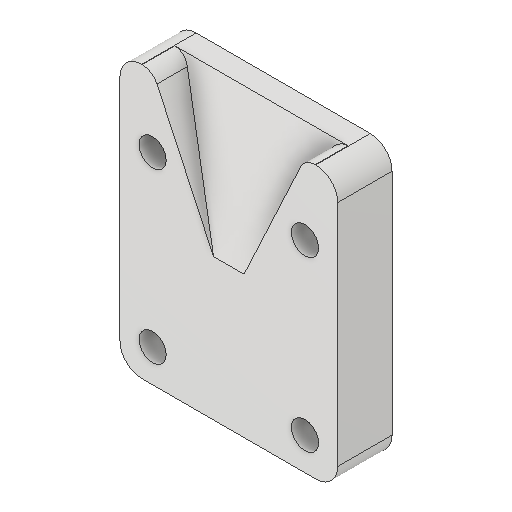
# Autodesk Inventor part: 3DP_PLA_Part_Detector_Top_Half
Saved by Autodesk Inventor 2025 (Build 290162010, 162A)
## iProperties
Created: 2018-07-20
Part Number: 3DP_PLA_Part_Detector_Top_Half
Material: ABS Plastic
Document SubType Name: Modeling
Designer: Andrzej
Density: 1.06 g/cm^3
Appearance: Smooth - White
Author: Andrzej
Autodesk Inventor part; units mm, degrees
ref_plane "YZ Plane" through (0, 0, 0) normal (1, 0, 0) x (0, 1, 0)
ref_plane "XZ Plane" through (0, 0, 0) normal (0, 1, 0) x (-1, 0, 0)
ref_plane "XY Plane" through (0, 0, 0) normal (0, 0, 1) x (1, 0, 0)
sketch "Sketch1" plane through (0, 0, 0) normal (0, 0, 1) x (1, 0, 0)
  line L0 (-9.6332, 12.3072) -> (10.3668, 12.3072)
  line L1 (10.3668, 12.3072) -> (10.3668, -12.6928)
  line L2 (10.3668, -12.6928) -> (-9.6332, -12.6928)
  line L3 (-9.6332, -12.6928) -> (-9.6332, 12.3072)
  line L4 (-4.3832, -2.6928) -> (5.1168, -2.6928)
  line L5 (5.1168, -2.6928) -> (5.1168, -7.7928)
  line L6 (5.1168, -7.7928) -> (-4.3832, -7.7928)
  line L7 (-4.3832, -7.7928) -> (-4.3832, -2.6928)
  line L8 (-1.0332, -2.6928) -> (-1.0332, -7.7928)
  line L9 (1.7668, -2.6928) -> (1.7668, -7.7928)
  line L10 (-1.0332, -2.6928) -> (-1.0332, 0.3072)
  line L11 (1.7668, -2.6928) -> (1.7668, 0.3072)
  line L12 (-1.0332, 0.3072) -> (-6.6332, 12.3072)
  line L13 (1.7668, 0.3072) -> (7.3668, 12.3072)
  line L14 (-1.0332, -7.7928) -> (-1.0332, -12.6928)
  line L15 (1.7668, -7.7928) -> (1.7668, -12.6928)
  point P0 (0, 0)
  dimension "d0" = 20
  dimension "d1" = 25
  dimension "d2" = 3.35
  dimension "d3" = 3.35
  dimension "d4" = 2.8
  dimension "d5" = 5.1
  dimension "d6" = 5.25
  dimension "d7" = 9.5
  dimension "d9" = 15
  dimension "d10" = 4.9
  dimension "d11" = 3
  dimension "d12" = 3
  dimension "d13" = 3
  dimension "d14" = 3
  constraints: 32 end point, 8 point on line, 5 parallel, 5 perpendicular, 2 horizontal, 2 vertical
  measures "d0" distance of L1.end L2.end
  measures "d1" distance of L0.end L1.end
  measures "d2" distance between parallel lines of L8 L7
  measures "d3" distance between parallel lines of L5 L9
  measures "d4" distance between parallel lines of L9 L8
  measures "d5" distance of L6.end L4.start
  measures "d6" distance between parallel lines of L3 L7
  measures "d7" distance between parallel lines of L5 L7
  measures "d9" distance between parallel lines of L0 L4
  measures "d10" distance between parallel lines of L2 L6
  measures "d11" distance from line of L3 L12.end
  measures "d12" distance from line of L1 L13.end
  measures "d13" distance of L8.start L10.end
  measures "d14" distance of L9.start L11.end
extrude "Extrusion1" add sketch "Sketch1" along normal blind 3 contours L0 L12 L10 L4 L7 L6 L14 L2 L3 | L0 L1 L2 L15 L6 L5 L4 L11 L13
extrude "Extrusion2" add sketch "Sketch1" against normal blind 5
chamfer "Chamfer1" distance 12 distance2 3 1 edges at (0.3668, 12.3072, 0) measured on face at (0.3668, 11.8072, 0)
sketch "Sketch3" plane through (0, 0, 3) normal (0, 0, 1) x (1, 0, 0)
  line L0 (-9.6332, 12.3072) -> (-9.6332, -12.6928) projected
  line L1 (-9.6332, -12.6928) -> (-1.0332, -12.6928) projected
  line L2 (-1.0332, -12.6928) -> (-1.0332, -7.7928) projected
  line L3 (-1.0332, -7.7928) -> (-4.3832, -7.7928) projected
  line L4 (-4.3832, -7.7928) -> (-4.3832, -2.6928) projected
  line L5 (-4.3832, -2.6928) -> (-1.0332, -2.6928) projected
  line L6 (-1.0332, -2.6928) -> (-1.0332, 0.3072) projected
  line L7 (-1.0332, 0.3072) -> (-6.6332, 12.3072) projected
  line L8 (-6.6332, 12.3072) -> (-9.6332, 12.3072) projected
  line L9 (10.3668, -12.6928) -> (10.3668, 12.3072) projected
  line L10 (10.3668, 12.3072) -> (7.3668, 12.3072) projected
  line L11 (7.3668, 12.3072) -> (1.7668, 0.3072) projected
  line L12 (1.7668, 0.3072) -> (1.7668, -2.6928) projected
  line L13 (1.7668, -2.6928) -> (5.1168, -2.6928) projected
  line L14 (5.1168, -2.6928) -> (5.1168, -7.7928) projected
  line L15 (5.1168, -7.7928) -> (1.7668, -7.7928) projected
  line L16 (1.7668, -7.7928) -> (1.7668, -12.6928) projected
  line L17 (1.7668, -12.6928) -> (10.3668, -12.6928) projected
  point P0 (0, 0)
  point P1 (-6.6332, 5.8072)
  point P2 (7.3668, 5.8072)
  point P3 (-6.6332, -9.6928)
  point P4 (7.3668, -9.6928)
  dimension "d24" = 25
  dimension "d25" = 6.5
  dimension "d26" = 3
  dimension "d27" = 4.9
  dimension "d28" = 3
  dimension "d29" = 3
  dimension "d37" = 5.25
  dimension "d38" = 3
  dimension "d39" = 3
  constraints: 2 horizontal alignment
  measures "d24" distance between parallel lines of L1 L8
  measures "d25" distance from line of L8 point (-6.633, 5.807)
  measures "d26" distance from line of L1 point (-6.633, -9.693)
  measures "d27" distance between parallel lines of L1 L3
  measures "d28" distance from line of L0 point (-6.633, 5.807)
  measures "d29" distance from line of L9 point (7.367, 5.807)
  measures "d37" distance between parallel lines of L0 L4
  measures "d38" distance from line of L0 point (-6.633, -9.693)
  measures "d39" distance from line of L9 point (7.367, -9.693)
hole "Hole1" at (-6.6332, 5.8072, 3) at (7.3668, 5.8072, 3) at (-6.6332, -9.6928, 3) at (7.3668, -9.6928, 3) direction (0, 0, -1) diameter 2.5 end through all
fillet "Fillet1" radius 1.5 2 edges at (-6.6332, 12.3072, 0) (7.3668, 12.3072, 0)
fillet "Fillet2" radius 2 4 edges at (-9.6332, 12.3072, -1) (10.3668, 12.3072, -1) (10.3668, -12.6928, -1) (-9.6332, -12.6928, -1)
sketch "Sketch4" plane through (0, 0, 3) normal (0, 0, 1) x (1, 0, 0)
  line L0 (-13.7185, 14.5378) -> (16.1134, 14.5378)
  line L1 (16.1134, 14.5378) -> (16.1134, -15.8403)
  line L2 (16.1134, -15.8403) -> (-13.7185, -15.8403)
  line L3 (-13.7185, -15.8403) -> (-13.7185, 14.5378)
  point P0 (0, 0)
  constraints: 8 end point, 2 parallel, 1 horizontal, 1 perpendicular
extrude "Extrusion4" cut sketch "Sketch4" against normal blind 3
equation "\"d3\" = d2"
equation "\"d6\" = -0.5 * d7 + 0.5 * d0"
equation "\"d12\" = d11"
equation "\"d14\" = d13"
equation "\"d29\" = d28"
equation "\"d39\" = d38"
body "Solid1"
